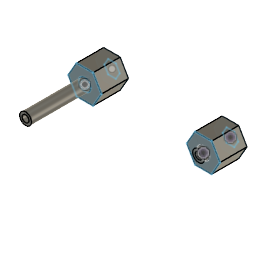
Final Connectors (Autodesk Fusion 360 design; units mm, degrees)
Autodesk Fusion 360 part; units mm, degrees
sketch "Sketch1" plane through (0, 0, 0) normal (0, 1, 0) x (1, 0, 0)
  line L0 (-7, 0) -> (-3.5, -6.0622)
  line L1 (-3.5, -6.0622) -> (3.5, -6.0622)
  line L2 (3.5, -6.0622) -> (7, 0)
  line L3 (7, 0) -> (3.5, 6.0622)
  line L4 (3.5, 6.0622) -> (-3.5, 6.0622)
  line L5 (-3.5, 6.0622) -> (-7, 0)
extrude "Extrude1" add sketch "Sketch1" along normal blind 11.43 makes body 1
sketch "Sketch2" plane through (0, 0, 0) normal (0, -1, 0) x (1, 0, 0)
  line L0 (-7, 0) -> (-3.5, -6.0622)
  line L1 (-3.5, -6.0622) -> (3.5, -6.0622)
  line L2 (3.5, -6.0622) -> (7, 0)
  line L3 (7, 0) -> (3.5, 6.0622)
  line L4 (3.5, 6.0622) -> (-3.5, 6.0622)
  line L5 (-3.5, 6.0622) -> (-7, 0)
  circle A0 centre (0, 0) radius 1.45
  circle A1 centre (0, 0) radius 2.5
  dimension "d3" = 2.9
  dimension "d4" = 5
  constraint coincident A0.centre A1.centre
  constraint concentric A0 A1
  measures "d3" diameter of A0
  measures "d4" diameter of A1
extrude "Extrude2" add sketch "Sketch2" along normal blind 2 contours A1 bodies 1
extrude "Extrude3" cut 1 faces at (1.0088, 0, 0.1932) along direction (0, 1, 0) blind 1 on bodies 1 bodies 1
sketch "Sketch3" plane through (0, 0, 0) normal (0, 1, 0) x (1, 0, 0)
  line L0 (-43, 0) -> (-46.5, 6.0622)
  line L1 (-46.5, 6.0622) -> (-53.5, 6.0622)
  line L2 (-53.5, 6.0622) -> (-57, 0)
  line L3 (-57, 0) -> (-53.5, -6.0622)
  line L4 (-53.5, -6.0622) -> (-46.5, -6.0622)
  line L5 (-46.5, -6.0622) -> (-43, 0)
  point P0 (-50, 0)
  point P1 (-50, 0)
  constraint coincident P0 P1
extrude "Extrude4" add sketch "Sketch3" along normal blind 11.43 separate body makes body 2
sketch "Sketch4" plane through (0, 0, 0) normal (0, -1, 0) x (1, 0, 0)
  line L0 (-43, 0) -> (-46.5, 6.0622)
  line L1 (-46.5, 6.0622) -> (-53.5, 6.0622)
  line L2 (-53.5, 6.0622) -> (-57, 0)
  line L3 (-57, 0) -> (-53.5, -6.0622)
  line L4 (-53.5, -6.0622) -> (-46.5, -6.0622)
  line L5 (-46.5, -6.0622) -> (-43, 0)
  circle A0 centre (-50, 0) radius 1.45
  circle A1 centre (-50, 0) radius 2.5
  dimension "d11" = 2.9
  dimension "d12" = 5
  constraint concentric A0 A1
  measures "d11" diameter of A0
  measures "d12" diameter of A1
sketch "Sketch5" plane through (0, 11.43, 0) normal (0, 1, 0) x (-1, 0, 0)
  line L0 (3.5, -6.0622) -> (7, 0)
  line L1 (7, 0) -> (3.5, 6.0622)
  line L2 (3.5, 6.0622) -> (-3.5, 6.0622)
  line L3 (-3.5, 6.0622) -> (-7, 0)
  line L4 (-7, 0) -> (-3.5, -6.0622)
  line L5 (-3.5, -6.0622) -> (3.5, -6.0622)
  line L6 (3.25, 0) -> (1.625, 2.8146)
  line L7 (1.625, 2.8146) -> (-1.625, 2.8146)
  line L8 (-1.625, 2.8146) -> (-3.25, 0)
  line L9 (-3.25, 0) -> (-1.625, -2.8146)
  line L10 (-1.625, -2.8146) -> (1.625, -2.8146)
  line L11 (1.625, -2.8146) -> (3.25, 0)
  dimension "d17" = 3.25
  measures "d17" distance of L6.start origin
extrude "Extrude7" cut sketch "Sketch5" against normal blind 3 contours L6 L7 L8 L9 L10 L11 bodies 1
sketch "Sketch6" plane through (0, 11.43, 0) normal (0, 1, 0) x (-1, 0, 0)
  line L0 (46.5, 6.0622) -> (43, 0)
  line L1 (43, 0) -> (46.5, -6.0622)
  line L2 (46.5, -6.0622) -> (53.5, -6.0622)
  line L3 (53.5, -6.0622) -> (57, 0)
  line L4 (57, 0) -> (53.5, 6.0622)
  line L5 (53.5, 6.0622) -> (46.5, 6.0622)
  line L6 (53.2, 0) -> (51.575, 2.8146)
  line L7 (51.575, 2.8146) -> (48.325, 2.8146)
  line L8 (48.325, 2.8146) -> (46.7, 0)
  line L9 (46.7, 0) -> (48.325, -2.8146)
  line L10 (48.325, -2.8146) -> (51.575, -2.8146)
  line L11 (51.575, -2.8146) -> (53.2, 0)
  point P0 (49.95, 0)
  dimension "d20" = 3.25
  measures "d20" distance of L6.start P0
extrude "Extrude8" cut sketch "Sketch6" against normal blind 3 contours L6 L7 L8 L9 L10 L11 bodies 2
extrude "Extrude9" add sketch "Sketch4" along normal blind 25 contours A1 bodies 2
extrude "Extrude10" cut sketch "Sketch4" against normal blind 3 contours A0 bodies 2
extrude "Extrude11" cut sketch "Sketch5" against normal blind 10 contours L6 L7 L8 L9 L10 L11 bodies 1
extrude "Extrude12" cut sketch "Sketch6" against normal blind 8 contours L6 L7 L8 L9 L10 L11 bodies 2
extrude "Extrude5" [suppressed]
extrude "Extrude6" [suppressed]
